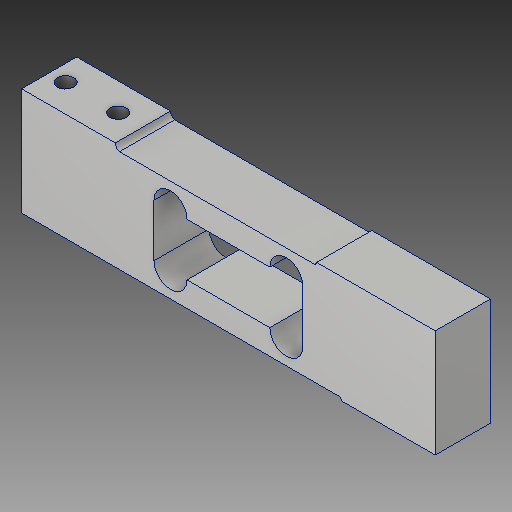
# Autodesk Inventor part: load cell
Saved by Autodesk Inventor 2018.1 (Build 221171000, 171)
## iProperties
Created: 2017-07-26
Part Number: load cell
Material: Aluminum 6061
Document SubType Name: Modeling
Designer: Tom
Density: 2.7 g/cm^3
Appearance: Aluminum - Flat
Mass: 234.476 g
Surface Area: 213.21 cm^2
Volume: 86.8429 cm^3
Author: Tom
Autodesk Inventor part; units mm, degrees
ref_plane "YZ Plane" through (0, 0, 0) normal (1, 0, 0) x (0, 1, 0)
ref_plane "XZ Plane" through (0, 0, 0) normal (0, 1, 0) x (-1, 0, 0)
ref_plane "XY Plane" through (0, 0, 0) normal (0, 0, 1) x (1, 0, 0)
sketch "Sketch1" plane through (0, 0, 0) normal (0, 0, 1) x (1, 0, 0)
  line L0 (0, 0) -> (150, 0) construction
  line L1 (150, 0) -> (150, 39) construction
  line L2 (150, 39) -> (0, 39) construction
  line L3 (0, 38) -> (150, 38) construction
  line L4 (0, 37) -> (150, 37) construction
  arc A0 (106.25, 37) -> (107, 38) centre (106.0005, 37.9684) ccw
  arc A1 (34, 39) -> (35.5, 37) centre (35.999, 38.9367) ccw
  line L5 (0, -1) -> (150, -1) construction
  arc A2 (116, -1) -> (115.25, 0) centre (115.0005, -0.9684) ccw
  line L6 (75, 37) -> (75, 0) construction
  line L7 (0, 18.5) -> (150, 18.5) construction
  line L8 (75, 28) -> (60, 28)
  arc A3 (60, 28) -> (48, 28) centre (54, 28) ccw
  line L9 (48, 28) -> (48, 18.5)
  line L10 (75, 28) -> (90, 28)
  arc A4 (102, 28) -> (90, 28) centre (96, 28) ccw
  line L11 (102, 28) -> (102, 18.5)
  line L12 (75, 9) -> (60, 9)
  arc A5 (48, 9) -> (60, 9) centre (54, 9) ccw
  line L13 (48, 9) -> (48, 18.5)
  arc A6 (90, 9) -> (102, 9) centre (96, 9) ccw
  line L14 (75, 9) -> (90, 9)
  line L15 (102, 9) -> (102, 18.5)
  line L16 (0, 39) -> (0, 0)
  line L17 (115.25, 0) -> (0, 0)
  line L18 (116, -1) -> (150, -1)
  line L19 (150, -1) -> (150, 38)
  line L20 (150, 38) -> (107, 38)
  line L21 (106.25, 37) -> (35.5, 37)
  line L22 (34, 39) -> (0, 39)
  dimension "d0" = 150
  dimension "d1" = 39
  dimension "d9" = 34
  dimension "d11" = 1
  dimension "d17" = 1
  dimension "d18" = 43
  dimension "d19" = 1.25
  dimension "d20" = 1
  dimension "d21" = 2.5
  dimension "d22" = 2
  dimension "d23" = 1
  dimension "d24" = 34
  dimension "d25" = 1.25
  dimension "d26" = 1
  dimension "d27" = 15
  dimension "d29" = 12
  dimension "d30" = 6
  constraints: 46 end point, 14 point on circle, 14 point on line, 11 symmetric about line, 7 centre point, 7 perpendicular, 4 collinear, 3 horizontal, 1 parallel, 1 vertical, 3 other
  measures "d0" distance of L2.end L1.end
  measures "d1" distance of L1.end L0.end
  measures "d9" distance of L2.end L22.start
  measures "d11" distance between parallel lines of L3 L2
  measures "d17" distance between parallel lines of L3 L4
  measures "d18" distance of L3.end L20.end
  measures "d19" distance of L20.end L21.start
  measures "d20" radius of A0
  measures "d21" distance of L22.start L21.end
  measures "d22" radius of A1
  measures "d23" distance between parallel lines of L0 L5
  measures "d24" distance of L5.end L18.start
  measures "d25" distance of L18.start L17.start
  measures "d26" radius of A2
  measures "d27" distance of L8.start L8.end
  measures "d29" distance of L8.end L9.start
  measures "d30" radius of A3
extrude "Extrusion1" add sketch "Sketch1" along normal blind 20
sketch "Sketch2" plane through (116, -1, 0) normal (0, -1, 0) x (1, 0, 0)
  line L0 (0, 20) -> (34, 20) construction
  line L1 (0, 0) -> (34, 0) construction
  line L2 (34, 0) -> (34, 20) construction
  line L3 (34, 20) -> (0, 20) construction
  line L4 (0, 20) -> (0, 0) construction
  circle A0 centre (9, 10) radius 3
  circle A1 centre (28.05, 10) radius 3
  line L5 (-116, 0) -> (-116, 20) construction
  line L6 (34, 0) -> (0, 0) construction
  line L7 (-116, 20) -> (34, 20) construction
  line L8 (34, 20) -> (34, 0) construction
  line L9 (34, 0) -> (-116, 0) construction
  line L10 (-116, 0) -> (-116, 20) construction
  line L11 (-116, 20) -> (-0.75, 20) construction
  dimension "d33" = 6
  dimension "d34" = 10
  dimension "d35" = 25
  dimension "d36" = 6
  dimension "d37" = 19.05
  constraints: 16 end point, 4 parallel, 2 centre point, 2 horizontal, 2 perpendicular
  measures "d33" diameter of A0
  measures "d34" distance from line of L0 A0.centre
  measures "d35" distance from line of L2 A0.centre
  measures "d36" diameter of A1
  measures "d37" distance of A1.centre A0.centre
extrude "Extrusion4" cut sketch "Sketch2" against normal blind 18
sketch "Sketch3" plane through (0, 39, 0) normal (0, 1, 0) x (1, 0, 0)
  line L0 (150, 0) -> (150, -20) construction
  line L1 (0, 0) -> (150, 0) construction
  line L2 (150, 0) -> (150, -20) construction
  line L3 (150, -20) -> (0, -20) construction
  line L4 (0, -20) -> (0, 0) construction
  circle A0 centre (5.95, -10) radius 3
  circle A1 centre (25, -10) radius 3
  dimension "d45" = 6
  dimension "d46" = 6
  dimension "d47" = 19.05
  dimension "d51" = 125
  dimension "d52" = 10
  dimension "d53" = 10
  constraints: 8 end point, 2 centre point, 2 parallel, 1 horizontal, 1 perpendicular
  measures "d45" diameter of A0
  measures "d46" diameter of A1
  measures "d47" distance of A1.centre A0.centre
  measures "d51" distance from line of L0 A1.centre
  measures "d52" distance from line of L1 A1.centre
  measures "d53" distance from line of L1 A0.centre
extrude "Extrusion5" cut sketch "Sketch3" against normal blind 18
thread "Thread1" size "M6x1" class "6H" standard "ANSI Metric M Profile" full length
thread "Thread2" size "M6x1" class "6H" standard "ANSI Metric M Profile" full length
thread "Thread3" size "M6x1" class "6H" standard "ANSI Metric M Profile" full length
thread "Thread4" size "M6x1" class "6H" standard "ANSI Metric M Profile" full length
equation "\"d0\" = lcl"
equation "\"d1\" = lch1"
equation "\"d9\" = lcwd2"
equation "\"d11\" = lch2 - lch1"
equation "\"d17\" = lch2 - lch1"
equation "\"d18\" = lcwd3"
equation "\"d23\" = lch2 - lch1"
equation "\"d24\" = lcwd2"
equation "\"d31\" = lcw"
equation "\"d33\" = dia1"
equation "\"d34\" = 0.5 * lcw"
equation "\"d35\" = lcwd1"
equation "\"d36\" = dia1"
equation "\"d37\" = lcsd"
equation "\"d43\" = td"
equation "\"d45\" = d48"
equation "\"d46\" = d48"
equation "\"d47\" = d49"
equation "\"d51\" = lcl - lcwd1"
equation "\"d52\" = 0.5 * lcw"
equation "\"d53\" = 0.5 * lcw"
equation "\"d54\" = td"
equation "\"dias\" = 8.8"
equation "\"stra1\" = 9.5"
equation "\"diab2\" = 6"
equation "\"stra\" = 25"
equation "\"db1\" = 6"
equation "\"ds1\" = 5.8"
equation "\"ds2\" = 1.6"
equation "\"ang\" = 120deg"
equation "\"db2\" = 3"
equation "\"diab3\" = 7"
equation "\"diab4\" = 3"
equation "\"dias1\" = 13.4375"
equation "\"dias3\" = 2"
equation "\"dias4\" = 4"
equation "\"t1\" = 3"
equation "\"t2\" = 3"
equation "\"t3\" = 6"
equation "\"t4\" = 6"
equation "\"t5\" = 3"
equation "\"diab1\" = 19"
equation "\"afw\" = 0.2"
equation "\"lcsd\" = 19.05"
equation "\"lcwd1\" = 25"
equation "\"lcwd2\" = 34"
equation "\"lcw\" = 20"
equation "\"lch1\" = 39"
equation "\"lch2\" = 40"
equation "\"lcl\" = 150"
equation "\"lcwd3\" = 43"
equation "\"dia1\" = 6"
equation "\"td\" = 18"
equation "\"d48\" = 6"
equation "\"d49\" = 19.05"
equation "\"bhh\" = 6"
equation "\"sw\" = 25"
equation "\"spacert\" = 2"
equation "\"sh\" = 31"
equation "\"pvct\" = 5"
equation "\"dia3\" = 8"
equation "\"dia4\" = 11"
equation "\"tankl\" = 379"
equation "\"play\" = 9"
equation "\"holeh\" = 26"
equation "\"surroundt\" = 5"
equation "\"slack\" = 0.5"
equation "\"play2\" = 3"
equation "\"diaoverflow\" = 25"
equation "\"diaph\" = 32"
equation "\"diawater\" = 25"
equation "\"diacucl\" = 32"
equation "\"diaair\" = 32"
equation "\"diasurroundhole\" = 42"
equation "\"diagrate\" = 12"
equation "\"gratespacing\" = 12.02082"
equation "\"bottomdist\" = 9.6355"
equation "\"sidedist\" = 13.9375"
equation "\"diahcl\" = 32"
equation "\"bracketwtop\" = 6"
equation "\"bracketwbottom\" = 6"
equation "\"nett\" = 1"
equation "\"nethole\" = 16"
equation "\"netside\" = 3.5"
equation "\"nettop\" = 7"
equation "\"netholespacing\" = 2"
equation "\"diaetape\" = 32"
body "Solid1"
